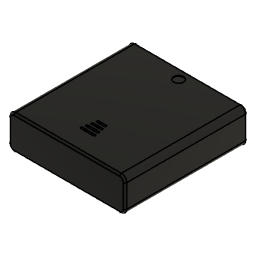
balancingRobot (Autodesk Fusion 360 archive; units mm, degrees)
design "AAbatteryHolder"
Autodesk Fusion 360 part; units mm, degrees
sketch "Sketch1" plane through (0, 0, 0) normal (0, 0, 1) x (1, 0, 0)
  line L0 (32.275, 33.915) -> (-32.275, 33.915)
  line L1 (-32.275, 33.915) -> (-32.275, -33.915)
  line L2 (-32.275, -33.915) -> (32.275, -33.915)
  line L3 (32.275, -33.915) -> (32.275, 33.915)
  line L4 (32.275, 33.915) -> (-32.275, -33.915) construction
  line L5 (-32.275, 33.915) -> (32.275, -33.915) construction
  circle A0 centre (0, 28.035) radius 2.73
  line L6 (-4, -21.665) -> (4, -21.665)
  line L7 (4, -21.665) -> (4, -22.665)
  line L8 (4, -22.665) -> (-4, -22.665)
  line L9 (-4, -22.665) -> (-4, -21.665)
  line L10 (4, -21.665) -> (-4, -22.665) construction
  line L11 (0, 0) -> (0, -33.915) construction
  line L12 (3.5, -19.165) -> (-3.5, -19.165)
  line L13 (-3.5, -19.165) -> (-3.5, -20.165)
  line L14 (-3.5, -20.165) -> (3.5, -20.165)
  line L15 (3.5, -20.165) -> (3.5, -19.165)
  line L16 (3.5, -19.165) -> (-3.5, -20.165) construction
  line L17 (-3.5, -19.165) -> (3.5, -20.165) construction
  line L18 (3, -16.665) -> (-3, -16.665)
  line L19 (-3, -16.665) -> (-3, -17.665)
  line L20 (-3, -17.665) -> (3, -17.665)
  line L21 (3, -17.665) -> (3, -16.665)
  line L22 (3, -16.665) -> (-3, -17.665) construction
  line L23 (-3, -16.665) -> (3, -17.665) construction
  line L24 (2.5, -14.165) -> (-2.5, -14.165)
  line L25 (-2.5, -14.165) -> (-2.5, -15.165)
  line L26 (-2.5, -15.165) -> (2.5, -15.165)
  line L27 (2.5, -15.165) -> (2.5, -14.165)
  line L28 (2.5, -14.165) -> (-2.5, -15.165) construction
  line L29 (-2.5, -14.165) -> (2.5, -15.165) construction
  line L30 (0, -205.75) -> (0, 209.25)
  point P0 (0, -22.165)
  point P1 (0, -19.665)
  point P2 (0, -17.165)
  point P3 (0, -14.665)
  dimension "d51" = 64.55
  dimension "d52" = 67.83
  dimension "d53" = 5.46
  dimension "d54" = 5.88
  dimension "d60" = 11.25
  dimension "d61" = 1
  dimension "d62" = 8
  dimension "d63" = 7
  dimension "d64" = 1
  dimension "d65" = 1.5
  dimension "d66" = 6
  dimension "d67" = 1
  dimension "d68" = 1.5
  dimension "d69" = 5
  dimension "d70" = 1
  dimension "d71" = 1.5
  constraint horizontal L0
  constraint perpendicular L0 L1
  constraint parallel L0 L2
  constraint parallel L1 L3
  constraint coincident L4 L11.start
  constraint coincident L5 L11.start
  constraint coincident L11.start origin
  constraint horizontal L6
  constraint vertical L7
  constraint horizontal L8
  constraint vertical L9
  constraint midpoint L10 P0
  constraint midpoint L2 L11.end
  constraint coincident P0 L11
  constraint horizontal L12
  constraint perpendicular L12 L13
  constraint parallel L12 L14
  constraint parallel L13 L15
  constraint coincident L16 P1
  constraint coincident L17 P1
  constraint coincident L11 P1
  constraint horizontal L18
  constraint perpendicular L18 L19
  constraint parallel L18 L20
  constraint parallel L19 L21
  constraint coincident L22 P2
  constraint coincident L23 P2
  constraint coincident L11 P2
  constraint horizontal L24
  constraint perpendicular L24 L25
  constraint parallel L24 L26
  constraint parallel L25 L27
  constraint coincident L28 P3
  constraint coincident L29 P3
  constraint coincident L11 P3
  measures "d51" distance of L1.end L2.end
  measures "d52" distance of L0.end L1.end
  measures "d53" diameter of A0
  measures "d54" distance of L0 A0.centre
  measures "d60" distance of L2 L8
  measures "d61" distance of L6.start L8.end
  measures "d62" distance of L7.end L8.end
  measures "d63" distance of L13.end L14.end
  measures "d64" distance of L12.end L13.end
  measures "d65" distance of L6 L14
  measures "d66" distance of L19.end L20.end
  measures "d67" distance of L18.end L19.end
  measures "d68" distance of L12 L20
  measures "d69" distance of L25.end L26.end
  measures "d70" distance of L24.end L25.end
  measures "d71" distance of L18 L26
extrude "Extrude1" add sketch "Sketch1" against normal blind 18.79
extrude "Extrude2" cut sketch "Sketch1" against normal blind 0.38 contours A0 L30 | A0 L30
extrude "Extrude3" add sketch "Sketch1" along normal blind 0.1 contours L6 L7 L8 L30 | L6 L8 L9 L30 | L24 L25 L26 L30 | L24 L26 L27 L30 | L12 L14 L15 L30 | L12 L13 L14 L30 | L18 L19 L20 L30 | L18 L20 L21 L30
fillet "Fillet1" radius 3 4 edges at (32.275, 0, -18.79) (32.275, 0, 0) (-32.275, 0, 0) (-32.275, 0, -18.79)
fillet "Fillet2" radius 1 2 faces at (9.7583, -33.915, -12.5267) (-9.7583, 33.915, -12.5267)
